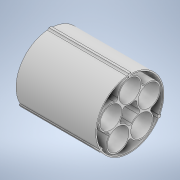
# Autodesk Inventor part: Engine
Saved by Autodesk Inventor 2020 (Build 240168000, 168)
## iProperties
Created: 2022-02-05
Part Number: Engine
Material: Generisch
Document SubType Name: Modeling
Designer: sp
Density: 1 g/cm^3
Appearance: Vorgabe
Author: sp
Autodesk Inventor part; units mm, degrees
ref_plane "YZ Plane" through (0, 0, 0) normal (1, 0, 0) x (0, 1, 0)
ref_plane "XZ Plane" through (0, 0, 0) normal (0, 1, 0) x (-1, 0, 0)
ref_plane "XY Plane" through (0, 0, 0) normal (0, 0, 1) x (1, 0, 0)
sketch "Skizze1" plane through (0, 0, 0) normal (1, 0, 0) x (0, 1, 0)
  circle A0 centre (0, 0) radius 30 construction
  circle A1 centre (17.5, 0) radius 9.5
  circle A2 centre (17.5, 0) radius 10.5
  circle A3 centre (5.4078, 16.6435) radius 9.5
  circle A4 centre (5.4078, 16.6435) radius 10.5
  circle A5 centre (-14.1578, 10.2862) radius 9.5
  circle A6 centre (-14.1578, 10.2862) radius 10.5
  circle A7 centre (-14.1578, -10.2862) radius 9.5
  circle A8 centre (-14.1578, -10.2862) radius 10.5
  circle A9 centre (5.4078, -16.6435) radius 9.5
  circle A10 centre (5.4078, -16.6435) radius 10.5
  circle A11 centre (0, 0) radius 4
  circle A12 centre (0, 0) radius 30
  circle A13 centre (0, 0) radius 29
  dimension "d0" = 60
  dimension "d1" = 17.5
  dimension "d2" = 19
  dimension "d3" = 21
  dimension "d6" = 360
  dimension "d8" = 8
  dimension "d12" = 58
  constraints: 14 centre point, 14 coincident, 1 concentric, 31 other
  measures "d0" diameter of A0
  measures "d1" distance of point (0, 0) point (17.5, 0)
  measures "d2" diameter of A1
  measures "d3" diameter of A2
  measures "d8" diameter of A11
  measures "d12" diameter of A13
extrude "Extrusion1" add sketch "Skizze1" against normal mid plane 70 contours A2 A10 A4 | A4 A2 | A2 A4 A6 | A10 A8 A2 | A2 A10 | A6 A8 A4 | A4 A6 | A10 A8 A6 | A8 A10 | A8 A6
fillet "Rundung1" radius 2 10 edges at (0, 13.1592, -9.5607) (0, -5.0264, -15.4696) (0, -16.2657, 0) (0, -5.0264, 15.4696) (0, 13.1592, 9.5607) (0, 9.7486, -7.0828) (0, 9.7486, 7.0828) (0, -3.7236, 11.4601) (0, -12.0499, 0) (0, -3.7236, -11.4601)
sketch "Skizze2" plane through (35, 0, 0) normal (1, 0, 0) x (0, 0, -1)
  circle A0 centre (0, 0) radius 30
  circle A1 centre (0, 0) radius 29
  dimension "d13" = 60
  dimension "d14" = 58
  constraints: 2 centre point, 2 coincident
  measures "d13" diameter of A0
  measures "d14" diameter of A1
extrude "Extrusion2" add sketch "Skizze2" against normal blind 70
sketch "Skizze3" plane through (0, 0, 0) normal (1, 0, 0) x (0, 1, 0)
  line L0 (35.299, 0) -> (22.394, 0) construction
  line L1 (46.9219, 0) -> (-63.2802, 0) construction
  arc A0 (17.2478, -10.497) -> (17.2478, 10.497) centre (17.5, 0) ccw projected
  line L2 (27.9523, 1) -> (30.9523, 1)
  line L3 (30.9523, 1) -> (30.9523, -1)
  line L4 (30.9523, -1) -> (27.9523, -1)
  line L5 (27.9523, -1) -> (27.9523, 1)
  point P0 (0, 0)
  point P1 (29.9278, 0)
  dimension "d17" = 2
  dimension "d18" = 3
  constraints: 12 end point, 3 horizontal, 3 point on line, 2 parallel, 1 perpendicular, 1 point on circle, 1 other
  measures "d17" distance between parallel lines of L4 L2
  measures "d18" distance between parallel lines of L5 L3
extrude "Extrusion3" add sketch "Skizze3" against normal mid plane 70
pattern_circular "Runde Anordnung1" count 3 over 360 about axis through (-10, 0, 0) along (1, 0, 0) of "Extrusion3"
fillet "Rundung2" radius 2 1 edges at (0, 29.9833, 1)
